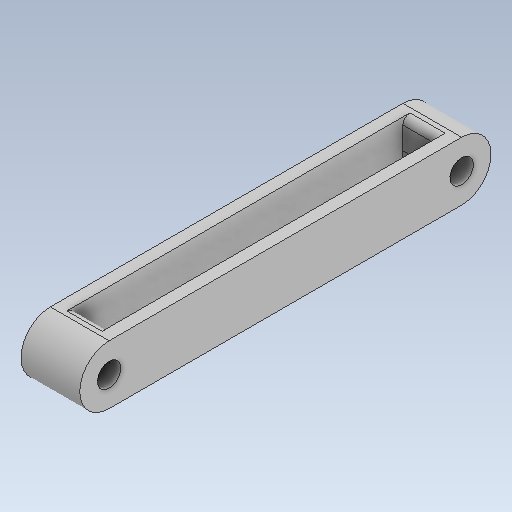
# Autodesk Inventor part: arm1
Saved by Autodesk Inventor 2020.3 (Build 243373000, 373)
## iProperties
Created: 2021-08-13
Part Number: arm1
Material: Generic
Document SubType Name: Modeling
Designer: 0x6f736f646f
Density: 1 g/cm^3
Appearance: Default
Mass: 395.832 g
Surface Area: 907.603 cm^2
Volume: 395.832 cm^3
Author: 0x6f736f646f
Autodesk Inventor part; units mm, degrees
ref_plane "YZ Plane" through (0, 0, 0) normal (1, 0, 0) x (0, 1, 0)
ref_plane "XZ Plane" through (0, 0, 0) normal (0, 1, 0) x (-1, 0, 0)
ref_plane "XY Plane" through (0, 0, 0) normal (0, 0, 1) x (1, 0, 0)
sketch "Sketch1" plane through (0, 0, 0) normal (1, 0, 0) x (0, 1, 0)
  circle A0 centre (0, 0) radius 25
  line L0 (0, 0) -> (0, 300)
  circle A1 centre (0, 300) radius 25
  circle A2 centre (0, 300) radius 10
  circle A3 centre (0, 0) radius 10
  line L1 (25, 300) -> (25, 0)
  line L2 (-25, 300) -> (-25, 0)
  dimension "d0" = 300
  dimension "d1" = 50
  dimension "d2" = 20
  constraints: 6 end point, 4 centre point, 4 point on circle, 3 tangent, 2 coincident, 2 equal radius, 2 vertical
  measures "d0" distance of L0.start L0.end
  measures "d1" diameter of A0
  measures "d2" diameter of A3
extrude "Extrusion1" add sketch "Sketch1" along normal blind 50
sketch "Sketch2" plane through (0, -25, 0) normal (0, -1, 0) x (1, 0, 0)
  line L0 (0, 0) -> (50, 0) projected
  line L1 (50, 300) -> (50, 0) projected
  line L2 (0, 0) -> (50, 0)
  line L3 (50, 0) -> (50, 300)
  line L4 (50, 300) -> (0, 300)
  line L5 (0, 300) -> (0, 0)
  line L6 (10, 10) -> (40, 10)
  line L7 (40, 10) -> (40, 290)
  line L8 (40, 290) -> (10, 290)
  line L9 (10, 290) -> (10, 10)
  dimension "d6" = 10
  constraints: 16 end point, 4 parallel, 2 perpendicular, 1 horizontal, 3 other
  measures "d6" distance between parallel lines of L5 L9
extrude "Extrusion2" cut sketch "Sketch2" against normal through all contours L9 L8 L7 L6
fillet "Fillet1" radius 6 4 edges at (25, 25, 290) (25, 25, 10) (25, -25, 10) (25, -25, 290)
body "Solid1"
